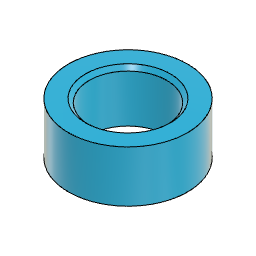
entretoise_dessus_arbre_secondaire_KOSMOS3-0 (Autodesk Fusion 360 design; units mm, degrees)
Autodesk Fusion 360 part; units mm, degrees
sketch "Esquisse1" plane through (0, 0, 0) normal (0, 0, 1) x (1, 0, 0)
  circle A0 centre (0, 0) radius 8
  circle A1 centre (0, 0) radius 5.2
  dimension "d1" = 10.4
  dimension "d2" = 16
  constraint coincident A0.centre A1.centre
  constraint concentric A0 A1
  measures "d1" diameter of A1
  measures "d2" diameter of A0
extrude "Extrusion1" add sketch "Esquisse1" along normal blind 6.9
chamfer "Chanfrein1" distance 0.5 angle 45 1 edges at (-4.8481, 1.8804, 6.9)
